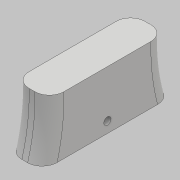
# Autodesk Inventor part: 支架滑塊4-15
Saved by Autodesk Inventor 2018 (Build 220112000, 112)
## iProperties
Created: 2021-04-15
Part Number: 支架滑塊4-15
Material: 一般
Document SubType Name: Modeling
Designer: 王鼎鈞
Density: 1 g/cm^3
Appearance: 預設
Author: 王鼎鈞
Autodesk Inventor part; units mm, degrees
ref_plane "YZ Plane" through (0, 0, 0) normal (1, 0, 0) x (0, 1, 0)
ref_plane "XZ Plane" through (0, 0, 0) normal (0, 1, 0) x (-1, 0, 0)
ref_plane "XY Plane" through (0, 0, 0) normal (0, 0, 1) x (1, 0, 0)
sketch "草圖1" plane through (0, 0, 0) normal (1, 0, 0) x (0, 1, 0)
  line L0 (0.5, 0) -> (8.5, 0)
  line L1 (9, 0) -> (9, -1)
  line L2 (9, -5) -> (0, -5)
  line L3 (0, -1) -> (0, 0)
  line L4 (4.5, 0) -> (4.5, 5.0637)
  line L5 (8.5, 0) -> (0.5, 0)
  line L6 (0.5, 0) -> (0.5, -1)
  line L7 (8.5, -1) -> (8.5, 0)
  arc A0 (8.5, -1) -> (9, -5) centre (21.9657, -1.348) ccw
  arc A1 (0, -5) -> (0.5, -1) centre (-12.9657, -1.348) ccw
  dimension "d0" = 9
  dimension "d1" = 5
  dimension "d2" = 1
  dimension "d3" = 8
  constraints: 16 end point, 4 point on circle, 3 parallel, 2 centre point, 2 horizontal, 2 perpendicular, 1 midpoint, 1 symmetric about line, 1 vertical, 2 other
  measures "d0" distance of L2.start L2.end
  measures "d1" distance of L1.start L2.start
  measures "d2" distance of L0.end L7.start
  measures "d3" distance of L6.end L7.start
extrude "擠出1" add sketch "草圖1" along normal blind 2.4
sketch "草圖2" plane through (2.4, 0, 0) normal (1, 0, 0) x (0, 0, -1)
  circle A0 centre (4.25, 4.5) radius 0.25
  line L0 (5, 0) -> (5, 9) projected
  point P0 (0, 0)
  dimension "d6" = 0.5
  dimension "d7" = 0.75
  constraints: 1 centre point
  measures "d6" diameter of A0
  measures "d7" distance from line of L0 A0.centre
extrude "擠出2" cut sketch "草圖2" against normal blind 5
fillet "圓角1" radius 1 8 edges at (2.4, 8.5995, -3.0188) (2.4, 8.5, -0.5) (0, 8.5995, -3.0188) (0, 8.5, -0.5) (2.4, 0.5, -0.5) (2.4, 0.4005, -3.0188) (0, 0.5, -0.5) (0, 0.4005, -3.0188)
move faces "移動1" translate (0, 0, -1) faces at (1.6, 3.5, 0)
